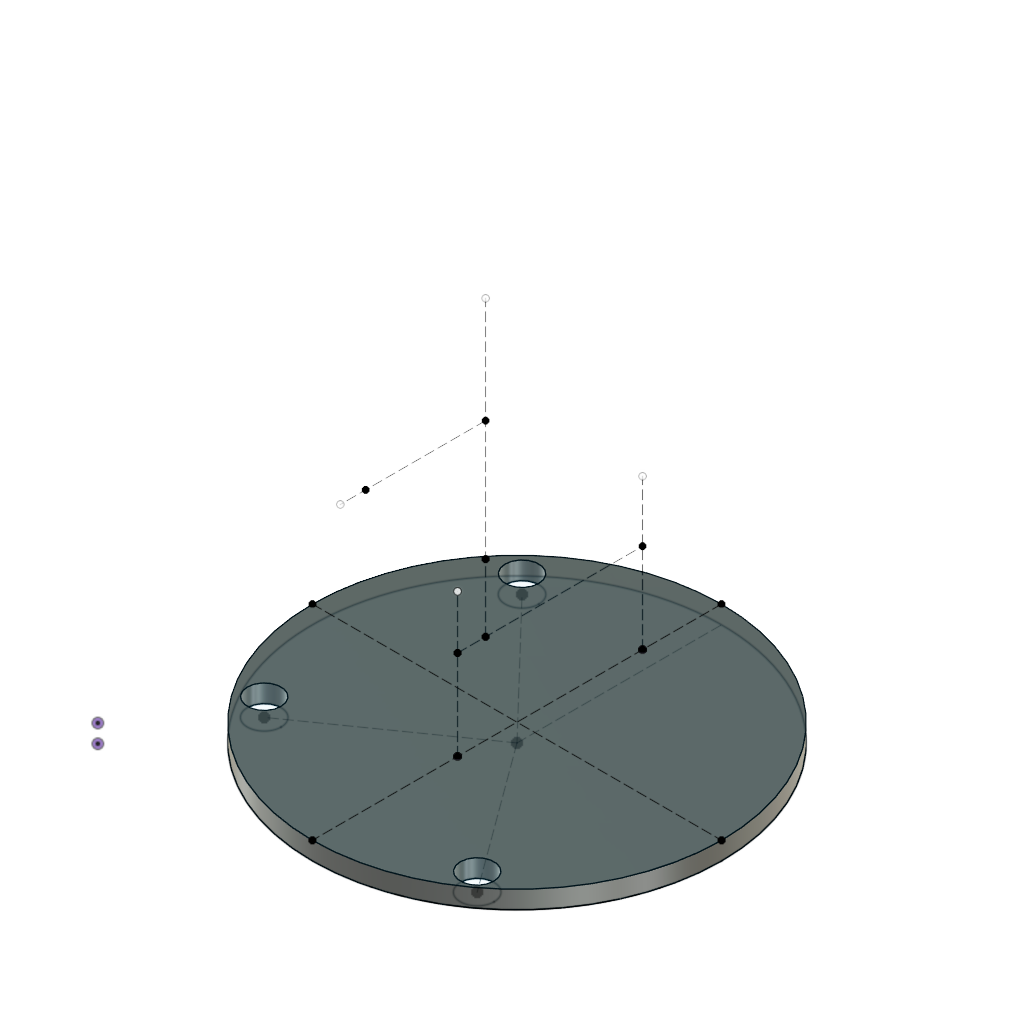
Adapterplatine (Autodesk Fusion 360 design; units mm, degrees)
Autodesk Fusion 360 part; units mm, degrees
sketch "Skizze1" plane through (0, 0, 0) normal (0, 0, 1) x (1, 0, 0)
  circle A0 centre (18.631, 18.76) radius 18.25
  circle A1 centre (7.381, 30.46) radius 1.5
  circle A2 centre (5.381, 9.46) radius 1.5
  circle A3 centre (28.381, 5.46) radius 1.5
  line L0 (18.631, 18.76) -> (7.381, 30.46) construction
  line L1 (18.631, 18.76) -> (5.381, 9.46) construction
  line L2 (18.631, 18.76) -> (28.381, 5.46) construction
  line L3 (18.631, 18.76) -> (18.631, 37.01) construction
  dimension "d1" = 36.5
  dimension "d4" = 18.631
  dimension "d5" = 18.76
  dimension "d6" = 3
  dimension "d7" = 7.381
  dimension "d8" = 30.46
  dimension "d9" = 9.46
  dimension "d10" = 5.381
  dimension "d11" = 5.46
  dimension "d12" = 28.381
  dimension "d24" = 43.877
  dimension "d25" = 125.065
  dimension "d26" = 143.756
  dimension "d27" = 16.2312
  dimension "d28" = 16.188
  dimension "d29" = 16.491
  constraint equal A1 A2
  constraint equal A1 A3
  constraint coincident A0.centre L0.start
  constraint coincident A1.centre L0.end
  constraint coincident A2.centre L1.end
  constraint coincident A3.centre L2.end
  constraint coincident A0 L3.end
  constraint vertical L3
  measures "d1" diameter of A0
  measures "d4" horizontal distance of origin A0.centre
  measures "d5" vertical distance of origin A0.centre
  measures "d6" diameter of A1
  measures "d7" horizontal distance of origin A1.centre
  measures "d8" vertical distance of origin A1.centre
  measures "d9" vertical distance of origin A2.centre
  measures "d10" horizontal distance of origin A2.centre
  measures "d11" vertical distance of origin A3.centre
  measures "d12" horizontal distance of origin A3.centre
  measures "d24" angle of L0 L3
  measures "d25" angle of L1 L3
  measures "d26" angle of L2 L3
  measures "d27" distance of A0.centre A1.centre
  measures "d28" distance of A0.centre A2.centre
  measures "d29" distance of A0.centre A3.centre
extrude "Extrusion1" add sketch "Skizze1" along normal blind 1.6
sketch "Skizze2" plane through (0, 0, 1.6) normal (0, 0, 1) x (-1, 0, 0)
  circle A0 centre (-5.381, -9.46) radius 1.5
  circle A1 centre (-7.381, -30.46) radius 1.5
  circle A2 centre (-28.381, -5.46) radius 1.5
  circle A3 centre (-18.631, -18.76) radius 18.25
  line L0 (-18.631, -37.01) -> (-18.631, -0.51) construction
  line L1 (-0.381, -18.76) -> (-36.881, -18.76) construction
  point P0 (-18.631, -29.96)
  point P1 (-18.631, -13.46)
  dimension "d13" = 13.46
  dimension "d15" = 29.96
  constraint coincident A3 L0.start
  constraint coincident A3 L0.end
  constraint vertical L0
  constraint coincident A3 L1.start
  constraint coincident A3 L1.end
  constraint horizontal L1
  constraint coincident A3.centre L1
  constraint coincident A3.centre L0
  constraint coincident L0 P1
  constraint coincident L0 P0
  measures "d13" vertical distance of origin P1
  measures "d15" vertical distance of origin P0
ref_plane "Arbeitsebene1" through (18.631, 0, 0) normal (1, 0, 0) x (0, 1, 0)
sketch "Skizze3" plane through (18.631, 0, 0) normal (1, 0, 0) x (0, 1, 0)
  line L0 (13.46, 1.6) -> (13.46, 14.3588) construction
  line L1 (29.96, 1.6) -> (29.96, 15) construction
  line L2 (13.46, 9.6) -> (29.96, 9.6) construction
  line L3 (15.96, 9.6) -> (15.96, 35.7478) construction
  line L4 (15.96, 26.3) -> (3, 26.3) construction
  point P0 (13.46, 1.6)
  point P1 (29.96, 1.6)
  point P2 (13.46, 9.6)
  point P3 (29.96, 9.6)
  point P4 (15.96, 9.6)
  point P5 (15.96, 15.6)
  point P6 (15.96, 26.3)
  point P7 (5.26, 26.3)
  dimension "d18" = 8
  dimension "d19" = 8
  dimension "d20" = 2.5
  dimension "d21" = 6
  dimension "d22" = 10.7
  dimension "d23" = 10.7
  constraint coincident P0 L0.start
  constraint vertical L0
  constraint coincident P1 L1.start
  constraint vertical L1
  constraint coincident L0 P2
  constraint coincident L1 P3
  constraint coincident P2 L2.start
  constraint coincident P3 L2.end
  constraint coincident L2 P4
  constraint coincident P4 L3.start
  constraint perpendicular L2 L3
  constraint coincident L3 P5
  constraint coincident L3 P6
  constraint coincident P6 L4.start
  constraint perpendicular L3 L4
  constraint coincident L4 P7
  measures "d18" distance of P0 P2
  measures "d19" distance of P1 P3
  measures "d20" distance of P2 P4
  measures "d21" distance of P4 P5
  measures "d22" distance of P5 P6
  measures "d23" distance of P6 P7
equation "d19 = d18"
